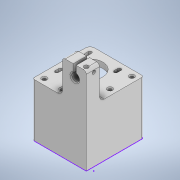
# Autodesk Inventor part: motor_holder_mirror
Saved by Autodesk Inventor 2021 (Build 250183000, 183)
## iProperties
Created: 2023-01-30
Part Number: motor_holder_mirror
Material: Типовые
Document SubType Name: Modeling
Designer: ignat
Density: 1 g/cm^3
Appearance: По умолчанию
Author: ignat
Autodesk Inventor part; units mm, degrees
ref_plane "YZ Plane" through (0, 0, 0) normal (1, 0, 0) x (0, 1, 0)
ref_plane "XZ Plane" through (0, 0, 0) normal (0, 1, 0) x (-1, 0, 0)
ref_plane "XY Plane" through (0, 0, 0) normal (0, 0, 1) x (1, 0, 0)
sketch "Эскиз1" plane through (0, 0, 0) normal (0, 1, 0) x (-1, 0, 0)
  circle A0 centre (0, 0) radius 1.75
  circle A1 centre (-2.25, -27.25) radius 1.75
  circle A2 centre (-27.25, -2.25) radius 1.75
  line L0 (4, 4) -> (-52.5, 4)
  line L1 (4, 4) -> (4, -56.5)
  line L2 (-8.5, -50.25) -> (-8.5, -10.5)
  line L3 (-10.5, -8.5) -> (-46.25, -8.5)
  arc A3 (-8.5, -10.5) -> (-10.5, -8.5) centre (-10.5, -10.5) ccw
  line L4 (4, -56.5) -> (-2.25, -56.5)
  arc A4 (-8.5, -50.25) -> (-2.25, -56.5) centre (-2.25, -50.25) ccw
  circle A5 centre (-2.25, -50.25) radius 1.75
  line L5 (-52.5, 4) -> (-52.5, -2.25)
  arc A6 (-52.5, -2.25) -> (-46.25, -8.5) centre (-46.25, -2.25) ccw
  circle A7 centre (-46.25, -2.25) radius 1.75
  point P0 (-8.5, -56.5)
  point P1 (-52.5, -8.5)
  dimension "d3" = 2
  dimension "d23" = 6.25
  dimension "d25" = 6.25
  constraints: 12 end point, 8 centre point, 6 point on circle, 6 tangent, 4 point on line, 2 coincident, 2 horizontal, 2 vertical, 1 parallel, 1 perpendicular
  measures "d3" radius of A3
  measures "d23" radius of A4
  measures "d25" radius of A6
extrude "Выдавливание1" add sketch "Эскиз1" along normal blind 50
sketch "Эскиз2" plane through (0, 50, 0) normal (0, 1, 0) x (1, 0, 0)
  arc A0 (13.25, 15) -> (16.75, 15) centre (15, 15) ccw
  arc A1 (13.25, 46) -> (16.75, 46) centre (15, 46) ccw
  arc A2 (44.25, 15) -> (47.75, 15) centre (46, 15) ccw
  arc A3 (44.25, 46) -> (47.75, 46) centre (46, 46) ccw
  arc A4 (17, 30.5) -> (44, 30.5) centre (30.5, 30.5) ccw
  arc A5 (16.75, 19) -> (13.25, 19) centre (15, 19) ccw
  arc A6 (16.75, 50) -> (13.25, 50) centre (15, 50) ccw
  arc A7 (47.75, 19) -> (44.25, 19) centre (46, 19) ccw
  arc A8 (47.75, 50) -> (44.25, 50) centre (46, 50) ccw
  arc A9 (44, 34.5) -> (17, 34.5) centre (30.5, 34.5) ccw
  line L0 (13.25, 15) -> (13.25, 19)
  line L1 (13.25, 46) -> (13.25, 50)
  line L2 (16.75, 50) -> (16.75, 46)
  line L3 (16.75, 19) -> (16.75, 15)
  line L4 (47.75, 15) -> (47.75, 19)
  line L5 (44.25, 19) -> (44.25, 15)
  line L6 (44.25, 46) -> (44.25, 50)
  line L7 (47.75, 50) -> (47.75, 46)
  line L8 (44, 30.5) -> (44, 34.5)
  line L9 (17, 30.5) -> (17, 34.5)
  line L10 (52.5, 51.5) -> (52.5, -4)
  line L11 (47.5, 56.5) -> (-4, 56.5)
  line L12 (-4, 56.5) -> (-4, -4) projected
  line L13 (-4, 56.5) -> (-4, -4)
  line L14 (-4, -4) -> (52.5, -4)
  arc A10 (52.5, 51.5) -> (47.5, 56.5) centre (47.5, 51.5) ccw
  circle A11 centre (46.25, 2.25) radius 1.75 projected
  circle A12 centre (27.25, 2.25) radius 1.75 projected
  circle A13 centre (0, 0) radius 1.75 projected
  circle A14 centre (2.25, 27.25) radius 1.75 projected
  circle A15 centre (2.25, 50.25) radius 1.75 projected
  point P0 (-4, 56.5)
  constraints: 28 end point, 22 point on circle, 11 centre point, 8 point on line, 8 tangent, 2 equal length, 2 perpendicular
extrude "Выдавливание2" add sketch "Эскиз2" along normal blind 6
chamfer "Фаска1" distance 1 angle 45 4 edges at (44.5, 56, -2.25) (25.5, 56, -2.25) (0.5, 56, -27.25) (0.5, 56, -50.25)
fillet "Сопряжение1" radius 2 2 edges at (52.5, 28, 4) (-4, 28, -56.5)
sketch "Эскиз3" plane through (0, 56, 0) normal (0, 1, 0) x (1, 0, 0)
  line L0 (-4, -4) -> (21, -4)
  line L1 (21, -4) -> (21, 10)
  line L2 (21, 10) -> (-4, 10)
  line L3 (-4, 10) -> (-4, -4)
  circle A0 centre (0, 0) radius 1.75 projected
  dimension "d30" = 25
  dimension "d31" = 14
  dimension "d48" = 4
  dimension "d49" = 4
  constraints: 8 end point, 2 parallel, 1 horizontal, 1 perpendicular
  measures "d30" distance of L2.end L1.end
  measures "d31" distance of L1.end L0.end
  measures "d48" horizontal distance of point (0, 0) L0.start
  measures "d49" horizontal distance of L0.start point (0, 0)
extrude "Выдавливание3" add sketch "Эскиз3" along normal blind 35
fillet "Сопряжение2" radius 5 2 edges at (21, 56, -3) (8.5, 56, -10)
sketch "Эскиз4" plane through (-4, 61, -10) normal (0, 0, -1) x (-1, 0, 0)
  arc A0 (-13.5, 21.8158) -> (-10.5, 21.8158) centre (-12, 18) ccw
  line L0 (-13.5, 21.8158) -> (-13.5, 30)
  line L1 (-13.5, 30) -> (-10.5, 30)
  line L2 (-10.5, 30) -> (-10.5, 21.8158)
  point P0 (-4, -61)
  dimension "d38" = 8.2
  constraints: 6 end point, 2 point on circle, 1 centre point, 1 horizontal, 1 perpendicular, 1 vertical
  measures "d38" diameter of A0
extrude "Выдавливание4" cut sketch "Эскиз4" against normal through all
sketch "Эскиз5" plane through (21, 91, 4) normal (1, 0, 0) x (0, 0, -1)
  circle A0 centre (8, -5) radius 1.75
  line L0 (0, 7.5329) -> (2, 7.5329)
  point P0 (4, -91)
  dimension "d45" = 3.5
  dimension "d50" = 2
  constraints: 2 end point, 1 centre point, 1 horizontal
  measures "d45" diameter of A0
  measures "d50" distance of L0.start L0.end
extrude "Выдавливание5" cut sketch "Эскиз5" against normal through all
sketch "Эскиз6" plane through (0, 91, 0) normal (0, 1, 0) x (1, 0, 0)
  circle A0 centre (0, 0) radius 2.25
  dimension "d51" = 4.5
  constraints: 1 centre point, 1 coincident
  measures "d51" diameter of A0
extrude "Выдавливание6" cut sketch "Эскиз6" against normal blind 15
chamfer "Фаска2" distance 2 angle 45 1 edges at (21, 86, -2.25)
fillet "Сопряжение4" radius 3 4 edges at (21, 91, -3) (-4, 91, -3) (22.4645, 57.4645, -11.4645) (21, 76, -10)
chamfer "Фаска3" distance 1 angle 45 2 edges at (8, 74.9, -10) (8, 74.9, 4)
sketch "Эскиз7" plane through (0, 56, 0) normal (0, 1, 0) x (1, 0, 0)
  arc A0 (13.25, 15) -> (16.75, 15) centre (15, 15) ccw projected
  circle A1 centre (15, 15) radius 3.5
  point P0 (0, 0)
  dimension "d61" = 7
  constraints: 1 centre point, 1 coincident
  measures "d61" diameter of A1
extrude "Выдавливание7" cut sketch "Эскиз7" along normal blind 15
mirror "Зеркальное отражение1" about plane through (-4, 0, -56.5) normal (-1, 0, 0) remove original yes
sketch "Эскиз8" plane through (-58.5, 0, 4) normal (0, -1, 0) x (1, 0, 0)
  arc A0 (52.5, -60.5) -> (54.5, -58.5) centre (52.5, -58.5) ccw
  line L0 (54.5, -58.5) -> (54.5, 0)
  line L1 (54.5, 0) -> (0, 0)
  arc A1 (0, 0) -> (-2, -2) centre (0, -2) ccw
  line L2 (-2, -2) -> (-2, -6.25)
  arc A2 (-2, -6.25) -> (4.25, -12.5) centre (4.25, -6.25) ccw
  line L3 (4.25, -12.5) -> (40, -12.5)
  arc A3 (42, -14.5) -> (40, -12.5) centre (40, -14.5) ccw
  line L4 (42, -14.5) -> (42, -54.25)
  arc A4 (42, -54.25) -> (48.25, -60.5) centre (48.25, -54.25) ccw
  line L5 (48.25, -60.5) -> (52.5, -60.5)
  circle A5 centre (48.25, -31.25) radius 1.75
  circle A6 centre (50.5, -4) radius 1.75
  circle A7 centre (23.25, -6.25) radius 1.75
  circle A8 centre (4.25, -6.25) radius 1.75
  circle A9 centre (48.25, -54.25) radius 1.75
  point P0 (58.5, -4)
  constraints: 19 centre point, 12 end point, 10 point on circle
